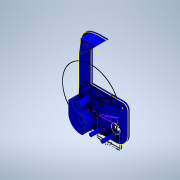
# Autodesk Inventor part: end carp left
Saved by Autodesk Inventor 2022 (Build 260153000, 153)
## iProperties
Created: 2022-12-27
Part Number: end carp left
Material: Типовые
Document SubType Name: Modeling
Designer: akapu
Density: 1 g/cm^3
Appearance: По умолчанию
Author: akapu
Autodesk Inventor part; units mm, degrees
sketch "Эскиз1" plane through (0, 0, 0) normal (0, 0, 1) x (1, 0, 0)
  line L0 (177.53, 10) -> (177.53, -9.022) projected
  line L1 (177.53, -9.022) -> (165.53, -9.022) projected
  line L2 (165.53, -9.022) -> (165.53, 10) projected
  line L3 (165.53, 10) -> (177.53, 10) projected
  line L4 (165.53, -76) -> (165.53, -56.978) projected
  line L5 (165.53, -56.978) -> (177.53, -56.978) projected
  line L6 (177.53, -56.978) -> (177.53, -76) projected
  line L7 (177.53, -76) -> (165.53, -76) projected
  circle A0 centre (170.53, -49.23) radius 1.6 projected
  circle A1 centre (170.53, -16.77) radius 1.6 projected
  line L8 (181.53, -107.5) -> (181.53, 41.5) projected
  spline S0 degree 3 poles (170.4742, 56) (180.336, 55.2175) (180.2172, 51.2995) (181.53, 41.5) knots -0.786777 -0.786777 -0.786777 -0.786777 0 0 0 0 projected
  line L9 (7.0558, 56) -> (170.4742, 56) projected
  spline S1 degree 3 poles (7.0558, 56) (-2.806, 55.2175) (-2.6872, 51.2995) (-4, 41.5) knots -0.786777 -0.786777 -0.786777 -0.786777 0 0 0 0 projected
  line L10 (-4, 41.5) -> (-4, -107.5) projected
  spline S2 degree 3 poles (7.0558, -122) (-2.806, -121.2175) (-2.6872, -117.2995) (-4, -107.5) knots -0.786777 -0.786777 -0.786777 -0.786777 0 0 0 0 projected
  line L11 (170.4742, -122) -> (7.0558, -122) projected
  spline S3 degree 3 poles (170.4742, -122) (180.336, -121.2175) (180.2172, -117.2995) (181.53, -107.5) knots -0.786777 -0.786777 -0.786777 -0.786777 0 0 0 0 projected
  arc A2 (153.53, -93) -> (156.53, -96) centre (156.53, -93) ccw projected
  line L12 (156.53, -96) -> (174.53, -96) projected
  line L13 (174.53, -96) -> (174.53, -113) projected
  arc A3 (171.53, -116) -> (174.53, -113) centre (171.53, -113) ccw projected
  line L14 (171.53, -116) -> (6, -116) projected
  arc A4 (3, -113) -> (6, -116) centre (6, -113) ccw projected
  line L15 (3, -113) -> (3, -96) projected
  line L16 (3, -96) -> (21, -96) projected
  arc A5 (21, -96) -> (24, -93) centre (21, -93) ccw projected
  line L17 (24, -93) -> (24, 27) projected
  arc A6 (24, 27) -> (21, 30) centre (21, 27) ccw projected
  line L18 (21, 30) -> (3, 30) projected
  line L19 (3, 30) -> (3, 47) projected
  arc A7 (6, 50) -> (3, 47) centre (6, 47) ccw projected
  line L20 (6, 50) -> (171.53, 50) projected
  arc A8 (174.53, 47) -> (171.53, 50) centre (171.53, 47) ccw projected
  line L21 (174.53, 30) -> (174.53, 47) projected
  line L22 (174.53, 30) -> (156.53, 30) projected
  arc A9 (156.53, 30) -> (153.53, 27) centre (156.53, 27) ccw projected
  line L23 (153.53, 27) -> (153.53, -93) projected
  circle A10 centre (160.53, -81) radius 1.5 projected
  circle A11 centre (17, -81) radius 1.5 projected
  circle A12 centre (17, -51) radius 1.5 projected
  circle A13 centre (160.53, -51) radius 1.5 projected
  circle A14 centre (3, -81) radius 1.5 projected
  circle A15 centre (3, -51) radius 1.5 projected
  circle A16 centre (174.53, -81) radius 1.5 projected
  circle A17 centre (17, 15) radius 1.5 projected
  circle A18 centre (17, -15) radius 1.5 projected
  circle A19 centre (160.53, -15) radius 1.5 projected
  circle A20 centre (160.53, 15) radius 1.5 projected
  circle A21 centre (3, 15) radius 1.5 projected
  circle A22 centre (174.53, 15) radius 1.5 projected
  circle A23 centre (3, -15) radius 1.5 projected
  arc A24 (56.8183, -29.5099) -> (58.485, -27.5378) centre (56.485, -27.5378) ccw projected
  line L24 (58.485, -27.5378) -> (58.485, 14) projected
  arc A25 (61.485, 17) -> (58.485, 14) centre (61.485, 14) ccw projected
  line L25 (61.485, 17) -> (61.97, 17) projected
  arc A26 (61.97, 17) -> (64.97, 20) centre (61.97, 20) ccw projected
  line L26 (64.97, 27) -> (64.97, 20) projected
  arc A27 (64.97, 27) -> (61.97, 30) centre (61.97, 27) ccw projected
  line L27 (9.6271, 30) -> (61.97, 30) projected
  arc A28 (9.6271, 30) -> (-1.03, 20.7602) centre (9.8286, 19.0018) ccw projected
  line L28 (-1.03, 20.7602) -> (-1.03, 11.499) projected
  arc A29 (-1.03, 11.499) -> (0.1129, 8.6996) centre (2.97, 11.499) ccw projected
  arc A30 (0.97, 6.6) -> (0.1129, 8.6996) centre (-2.03, 6.6) ccw projected
  line L29 (0.97, 6.6) -> (0.97, -72.6) projected
  arc A31 (0.1129, -74.6996) -> (0.97, -72.6) centre (-2.03, -72.6) ccw projected
  arc A32 (0.1129, -74.6996) -> (-1.03, -77.499) centre (2.97, -77.499) ccw projected
  line L30 (-1.03, -77.499) -> (-1.03, -86.7602) projected
  arc A33 (-1.03, -86.7602) -> (9.6271, -96) centre (9.8286, -85.0018) ccw projected
  line L31 (61.97, -96) -> (9.6271, -96) projected
  arc A34 (61.97, -96) -> (64.97, -93) centre (61.97, -93) ccw projected
  line L32 (64.97, -86) -> (64.97, -93) projected
  arc A35 (64.97, -86) -> (61.97, -83) centre (61.97, -86) ccw projected
  line L33 (61.97, -83) -> (61.485, -83) projected
  arc A36 (58.485, -80) -> (61.485, -83) centre (61.485, -80) ccw projected
  line L34 (58.485, -80) -> (58.485, -48.5022) projected
  arc A37 (58.485, -48.5022) -> (56.8183, -46.5301) centre (56.485, -48.5022) ccw projected
  arc A38 (53.485, -45.3303) -> (56.8183, -46.5301) centre (58.485, -36.67) ccw projected
  arc A39 (52.485, -43.5982) -> (53.485, -45.3303) centre (54.485, -43.5982) ccw projected
  line L35 (52.485, -43.5982) -> (52.485, -32.4418) projected
  arc A40 (53.485, -30.7097) -> (52.485, -32.4418) centre (54.485, -32.4418) ccw projected
  arc A41 (56.8183, -29.5099) -> (53.485, -30.7097) centre (58.485, -39.37) ccw projected
  circle A42 centre (3, -81) radius 1.5 projected
  circle A43 centre (3, 15) radius 1.5 projected
  circle A44 centre (58.485, -89.515) radius 1.5 projected
  circle A45 centre (17, -51) radius 1.5 projected
  circle A46 centre (17, -15) radius 1.5 projected
  circle A47 centre (58.485, 23.515) radius 1.5 projected
  circle A48 centre (49.485, 22.73) radius 0.325 projected
  circle A49 centre (48.885, -25.77) radius 0.8 projected
  circle A50 centre (49.385, -32.52) radius 0.5 projected
  circle A51 centre (4.27, -36.27) radius 0.325 projected
  circle A52 centre (28.2, -73.38) radius 0.325 projected
  circle A53 centre (12.77, 15) radius 0.325 projected
  circle A54 centre (55.185, -49.79) radius 0.325 projected
  circle A55 centre (55.185, -4.51) radius 0.325 projected
  circle A56 centre (12.77, 22) radius 0.325 projected
  circle A57 centre (12.77, -88) radius 0.325 projected
  circle A58 centre (4.27, -23.42) radius 0.325 projected
  circle A59 centre (39.385, -40.52) radius 0.85 projected
  circle A60 centre (53.885, -25.77) radius 0.8 projected
  circle A61 centre (8.77, -88) radius 0.325 projected
  circle A62 centre (39.385, -35.52) radius 0.85 projected
  circle A63 centre (28.2, -60.76) radius 0.325 projected
  circle A64 centre (4.27, -47) radius 0.325 projected
  circle A65 centre (45.215, -90) radius 0.325 projected
  circle A66 centre (43.485, 24.73) radius 0.5 projected
  circle A67 centre (55.185, -69.03) radius 0.325 projected
  circle A68 centre (55.185, 15.73) radius 0.325 projected
  circle A69 centre (45.215, -83) radius 0.325 projected
  circle A70 centre (12.77, -81) radius 0.325 projected
  circle A71 centre (4.27, -8.84) radius 0.325 projected
  circle A72 centre (49.385, -43.52) radius 0.5 projected
  circle A73 centre (8.77, 22) radius 0.325 projected
  line L36 (6, 50) -> (12, 56)
  line L37 (3, 47) -> (3, 55.3611)
  circle A74 centre (3, 15) radius 7
  circle A75 centre (17, 15) radius 7
  line L38 (3, 8) -> (17, 8)
  circle A76 centre (3, 15) radius 2.6
  line L39 (3, 17.6) -> (24, 17.6)
  line L40 (5.6, 15) -> (7.6, 15)
  line L41 (7.6, 15) -> (7.6, 17.6)
  line L42 (7.6, 15) -> (7.6, 8)
  line L43 (7.6, 17.6) -> (20.4, 17.6)
  line L44 (20.4, 17.6) -> (20.4, 7.6)
  line L45 (20.4, 7.6) -> (7.6, 7.6)
  line L46 (7.6, 7.6) -> (7.6, 17.6)
  point P0 (0, 0)
  point P1 (23.4992, 17.6)
  point P2 (-4, 15)
  point P3 (10.5008, 17.6)
  point P4 (10, 15)
  point P5 (9.4992, 17.6)
  point P6 (24, 15)
  dimension "d8" = 5.2
  dimension "d15" = 2
  dimension "d16" = 12.8
  dimension "d17" = 10
  constraints: 22 end point, 5 point on line, 3 coincident, 3 parallel, 3 perpendicular, 3 vertical, 2 horizontal, 2 point on circle, 2 tangent, 1 centre point, 7 other
  measures "d8" diameter of A76
  measures "d15" distance of L40.start L40.end
  measures "d16" distance of L44.end L45.end
  measures "d17" distance of L43.end L44.end
extrude "Выдавливание1" add sketch "Эскиз1" along normal blind 1 contours L36 A7 L37 S1 L9 | L10 S1 L37 L19 L18 A28 L28 A74 | A74 L28 A29 A30 | A74 L39 A76 L40 L42 A30 A29 L28 | L28 A28 L18 A6 L17 L39 A75 A74 | L39 A75 A74 | A74 L42 L41 L39 | A74 L42 L38 | A75 L38 L42 A74 | A75 L39 L44 | L41 L40 A76 L39 | A75 L39 | A76 | L39 L17 A75 | A75 L44 L39 | A53 | A56 | A73
chamfer "Фаска1" distance 1 angle 45 1 edges at (15.5, 15, 1)
sketch "Эскиз2" plane through (0, 0, 1) normal (0, 0, 1) x (1, 0, 0)
  circle A0 centre (3, 15) radius 1.5 projected
  line L0 (24, 15) -> (24, 27) projected
  arc A1 (24, 27) -> (21, 30) centre (21, 27) ccw projected
  line L1 (21, 30) -> (3, 30) projected
  line L2 (3, 30) -> (3, 47) projected
  arc A2 (6, 50) -> (3, 47) centre (6, 47) ccw projected
  line L3 (6, 50) -> (12, 56) projected
  line L4 (12, 56) -> (7.0558, 56) projected
  line L5 (-4, 41.5) -> (-4, 15) projected
  arc A3 (-4, 15) -> (3, 8) centre (3, 15) ccw projected
  line L6 (3, 8) -> (17, 8) projected
  arc A4 (17, 8) -> (24, 15) centre (17, 15) ccw projected
  circle A5 centre (17, 15) radius 2.5 projected
  line L7 (3, 30) -> (3, 47) projected
  line L8 (3, 47) -> (3, 55.3611)
  arc A6 (6, 50) -> (3, 47) centre (6, 47) ccw projected
  circle A7 centre (3, 15) radius 1.5 projected
  line L9 (4.5, 15) -> (6.5, 15)
  line L10 (6.5, 15) -> (6.5, 16.5)
  line L11 (6.5, 16.5) -> (3, 16.5)
  line L12 (21, 30) -> (3, 30) projected
  line L13 (3, 16.5) -> (3, 30)
  circle A8 centre (3, 23.25) radius 1.6
  line L14 (6.5, 16.5) -> (19.3, 16.5)
  line L15 (19.3, 16.5) -> (19.3, 6.4)
  line L16 (19.3, 6.4) -> (6.5, 6.4)
  line L17 (6.5, 6.4) -> (6.5, 16.5)
  line L18 (19.3, 16.5) -> (19.3, 10)
  line L19 (19.3, 10) -> (19.3, 11.5)
  line L20 (19.3, 11.5) -> (6.5, 11.5)
  line L21 (12.9, 11.5) -> (16.15, 11.5)
  line L22 (16.15, 11.5) -> (9.65, 11.5)
  circle A9 centre (9.65, 11.5) radius 1
  circle A10 centre (16.15, 11.5) radius 1
  line L23 (19.3, 10) -> (6.5, 10)
  line L24 (9.65, 11.5) -> (18.15, 11.5)
  line L25 (18.172, 17.2) -> (6.5, 16.5)
  line L26 (17.4875, 20.5) -> (6.5, 16.5)
  arc A11 (18.1929, 16.5) -> (17.4875, 20.5) centre (6.5, 16.5) ccw
  line L27 (6.5, 16.5) -> (6.5, 16.7)
  line L28 (8.0036, 17.7621) -> (19.1448, 21.3116)
  circle A12 centre (3, 15) radius 2.6
  circle A13 centre (3, 23.25) radius 5.5
  line L29 (8.0036, 17.7621) -> (5.1102, 17.8522)
  line L30 (2.8349, 17.7525) -> (3.7176, 17.499)
  circle A14 centre (3, 23.25) radius 16.2607
  line L31 (6.5, 16.7) -> (18.172, 17.4)
  line L32 (6.5, 16.7) -> (3.7176, 17.499)
  line L33 (4.1923, 17.8808) -> (5.1102, 17.8522)
  line L34 (17.7935, 30) -> (3, 23.25)
  line L35 (3, 23.25) -> (18.9993, 26.1538)
  line L36 (21, 30) -> (3, 30) projected
  line L37 (18.9993, 26.1538) -> (8.3735, 28.8503)
  line L38 (18.9993, 26.1538) -> (3.8431, 30)
  circle A15 centre (3, 23.25) radius 6.75
  point P0 (0, 0)
  dimension "d41" = 11
  dimension "d23" = 2
  dimension "d24" = 3.2
  dimension "d25" = 12.8
  dimension "d26" = 10.1
  dimension "d27" = 6.5
  dimension "d28" = 1.5
  dimension "d29" = 3.25
  dimension "d30" = 6.5
  dimension "d31" = 2
  dimension "d32" = 2
  dimension "d35" = 8.5
  dimension "d39" = 0.2
  dimension "d40" = 5.2
  dimension "d42" = 16.572
  dimension "d44" = 14.239
  dimension "d45" = 24.526
  dimension "d48" = 24.526
  constraints: 58 end point, 11 point on line, 7 centre point, 7 coincident, 7 point on circle, 4 perpendicular, 4 tangent, 3 vertical, 2 midpoint, 2 parallel, 1 horizontal, 5 other
  measures "d23" distance of L9.start L9.end
  measures "d24" diameter of A8
  measures "d25" distance of L15.end L16.end
  measures "d26" distance of L14.end L15.end
  measures "d27" distance of L14.end L18.end
  measures "d28" distance of L18.end L19.end
  measures "d29" distance of L21.start L21.end
  measures "d30" distance of L21.end L22.end
  measures "d31" diameter of A9
  measures "d32" diameter of A10
  measures "d35" distance of L24.start L24.end
  measures "d39" distance of L27.end L27.start
  measures "d40" diameter of A12
  measures "d42" angle of L26 L25
  measures "d44" angle of L35 L34
  measures "d45" angle of L36 L34
  measures "d48" angle of L35 L37
sketch "Эскиз3" plane through (0, 0, 1) normal (0, 0, 1) x (1, 0, 0)
  arc A0 (-2.5, 23.25) -> (3, 17.75) centre (3, 23.25) ccw projected
  line L0 (3, 17.75) -> (3, 17.7051) projected
  line L1 (3, 17.7051) -> (6.5, 16.7) projected
  line L2 (6.5, 16.7) -> (18.172, 17.4) projected
  arc A1 (18.172, 17.4) -> (18.9993, 26.1538) centre (3, 23.25) ccw projected
  line L3 (18.9993, 26.1538) -> (4.6603, 29.7926) projected
  arc A2 (4.6603, 29.7926) -> (3, 30) centre (3, 23.25) ccw projected
  line L4 (3, 30) -> (3, 55.3611) projected
  spline S0 degree 3 poles (3, 55.3611) (-2.8051, 53.7936) (-2.8999, 49.7118) (-4, 41.5) knots -0.659309 -0.659309 -0.659309 -0.659309 0 0 0 0 projected
  line L5 (-4, 41.5) -> (-4, 23.25) projected
  line L6 (-4, 23.25) -> (-2.5, 23.25) projected
  circle A3 centre (3, 23.25) radius 1.6 projected
  line L7 (-2.331, 21.8972) -> (-3.7849, 21.5282)
  line L8 (-4, 41.5) -> (-4, 15) projected
  line L9 (-2.331, 21.8972) -> (-4, 21.4736)
  line L10 (-2.331, 21.8972) -> (-2.5249, 21.848)
  circle A4 centre (3, 23.25) radius 5.7
  circle A5 centre (3, 15) radius 2.6 projected
  line L11 (-2.5249, 21.848) -> (0.5844, 14.0383)
  arc A6 (-4, 15) -> (3, 8) centre (3, 15) ccw projected
  line L12 (3, 12.4) -> (3, 8)
  circle A7 centre (3, 10.2) radius 2.2
  line L13 (3, 30) -> (3, 55.3611) projected
  circle A8 centre (3, 15) radius 1.5 projected
  line L14 (24, 15) -> (24, 27) projected
  arc A9 (24, 27) -> (21, 30) centre (21, 27) ccw projected
  line L15 (21, 30) -> (3, 30) projected
  line L16 (3, 30) -> (3, 47) projected
  arc A10 (6, 50) -> (3, 47) centre (6, 47) ccw projected
  line L17 (6, 50) -> (12, 56) projected
  line L18 (12, 56) -> (7.0558, 56) projected
  spline S1 degree 3 poles (7.0558, 56) (-2.806, 55.2175) (-2.6872, 51.2995) (-4, 41.5) knots 0 0 0 0 1 1 1 1 projected
  line L19 (-4, 41.5) -> (-4, 15) projected
  arc A11 (-4, 15) -> (3, 8) centre (3, 15) ccw projected
  line L20 (3, 8) -> (17, 8) projected
  arc A12 (17, 8) -> (24, 15) centre (17, 15) ccw projected
  circle A13 centre (17, 15) radius 2.5 projected
  point P0 (0, 0)
  point P1 (-1.9767, 20.471)
  point P2 (-2.7, 23.25)
  point P3 (3, 8)
  dimension "d49" = 0.2
  constraints: 10 end point, 2 point on circle, 2 point on line, 1 coincident, 1 midpoint, 1 tangent, 1 vertical, 7 other
  measures "d49" distance of L7.start L10.end
extrude "Выдавливание2" add sketch "Эскиз3" along normal blind 5.8 contours A4 L11 A5 A7 A6 L8 L9 L7 | S1 L18 L17 A10 L4 | A7 L12 | L12 A7
ref_plane "РабПлоскость2" through (-3.5074, 8.5, 7.8) normal (0, 0, 1) x (1, 0, 0)
sketch "Эскиз4" plane through (0, 0, 1) normal (0, 0, 1) x (1, 0, 0)
  circle A0 centre (17, 15) radius 2.5 projected
  arc A1 (-2.5249, 21.848) -> (-1.9767, 20.471) centre (3, 23.25) ccw projected
  line L0 (-1.9767, 20.471) -> (0.5844, 14.0383) projected
  arc A2 (0.5844, 14.0383) -> (3, 12.4) centre (3, 15) ccw projected
  arc A3 (3, 8) -> (3, 12.4) centre (3, 10.2) ccw projected
  line L1 (3, 8) -> (17, 8) projected
  arc A4 (17, 8) -> (24, 15) centre (17, 15) ccw projected
  line L2 (24, 15) -> (24, 27) projected
  arc A5 (24, 27) -> (21, 30) centre (21, 27) ccw projected
  line L3 (21, 30) -> (3, 30) projected
  line L4 (3, 30) -> (3, 47) projected
  line L5 (3, 47) -> (3, 55.3611) projected
  line L6 (-4, 41.5) -> (-4, 21.4736) projected
  circle A6 centre (3, 15) radius 1.5 projected
  circle A7 centre (3, 23.25) radius 1.6 projected
  circle A8 centre (3, 23.25) radius 1.6
  line L7 (-4, 21.4736) -> (-2.5249, 21.848) projected
  circle A9 centre (3, 23.25) radius 1.45
  point P0 (0, 0)
  dimension "d58" = 2.9
  constraints: 2 centre point, 2 coincident, 1 concentric, 1 other
  measures "d58" diameter of A9
extrude "Выдавливание3" add sketch "Эскиз4" along normal up to surface (6.8 mm away) contours A9
sketch "Эскиз5" plane through (0, 0, 1) normal (0, 0, 1) x (1, 0, 0)
  circle A0 centre (9.65, 11.5) radius 1 projected
  circle A1 centre (16.15, 11.5) radius 1 projected
  circle A2 centre (9.65, 11.5) radius 0.95
  circle A3 centre (16.15, 11.5) radius 0.95
  point P0 (0, 0)
  dimension "d54" = 1.9
  dimension "d55" = 1.9
  constraints: 2 centre point, 2 coincident
  measures "d54" diameter of A2
  measures "d55" diameter of A3
ref_plane "РабПлоскость1" through (-3.5074, 8.5, 7.8) normal (0, 0, 1) x (1, 0, 0)
extrude "Выдавливание4" add sketch "Эскиз5" along normal up to surface (6.8 mm away) contours A2 | A3
sketch "Эскиз6" plane through (0, 0, 6.8) normal (0, 0, 1) x (1, 0, 0)
  line L0 (3, 47) -> (3, 55.3611) projected
  line L1 (6, 50) -> (12, 56) projected
  line L2 (3, 51.1805) -> (9.5279, 56)
  line L3 (12, 56) -> (7.0558, 56) projected
  circle A0 centre (6.264, 53.5903) radius 0.95
  point P0 (0, 0)
  dimension "d59" = 1.9
  constraints: 3 midpoint, 2 end point, 1 centre point
  measures "d59" diameter of A0
ref_plane "РабПлоскость3" through (-3.5074, 8.5, 7.8) normal (0, 0, 1) x (1, 0, 0)
extrude "Выдавливание5" add sketch "Эскиз6" along normal up to surface (1 mm away)
sketch "Эскиз7" plane through (0, 0, 1) normal (0, 0, 1) x (1, 0, 0)
  circle A0 centre (3, 15) radius 2.6 projected
  circle A1 centre (3, 15) radius 2.5
  line L0 (5.4951, 14.8437) -> (5.1957, 10.0625)
  arc A2 (3, 8) -> (3, 12.4) centre (3, 10.2) ccw projected
  circle A3 centre (3, 23.25) radius 1.45 projected
  arc A4 (-2.5249, 21.848) -> (-1.9767, 20.471) centre (3, 23.25) ccw projected
  circle A5 centre (3, 23.25) radius 5.7
  line L1 (2.3734, 17.5845) -> (3.2748, 17.4848)
  circle A6 centre (9.65, 11.5) radius 0.95 projected
  circle A7 centre (16.15, 11.5) radius 0.95 projected
  circle A8 centre (3, 23.25) radius 1.45 projected
  circle A9 centre (17, 15) radius 2.5 projected
  line L2 (3, 47) -> (3, 55.3611) projected
  line L3 (-4, 41.5) -> (-4, 21.4736) projected
  line L4 (-4, 21.4736) -> (-2.5249, 21.848) projected
  arc A10 (-2.5249, 21.848) -> (-1.9767, 20.471) centre (3, 23.25) ccw projected
  line L5 (-1.9767, 20.471) -> (0.5844, 14.0383) projected
  arc A11 (0.5844, 14.0383) -> (3, 12.4) centre (3, 15) ccw projected
  arc A12 (3, 8) -> (3, 12.4) centre (3, 10.2) ccw projected
  line L6 (3, 8) -> (17, 8) projected
  arc A13 (17, 8) -> (24, 15) centre (17, 15) ccw projected
  line L7 (24, 15) -> (24, 27) projected
  arc A14 (24, 27) -> (21, 30) centre (21, 27) ccw projected
  line L8 (21, 30) -> (3, 30) projected
  line L9 (3, 30) -> (3, 47) projected
  circle A15 centre (3, 15) radius 1.5 projected
  point P0 (0, 0)
  point P1 (-1.9767, 20.471)
  dimension "d62" = 5
  constraints: 5 point on circle, 4 end point, 4 tangent, 2 centre point, 2 coincident, 2 other
  measures "d62" diameter of A1
extrude "Выдавливание6" add sketch "Эскиз7" along normal up to surface (5.8 mm away) contours A0 L1 A1 L0 | L5 A5 L1 A0 | A0 L0 A2 | A1
